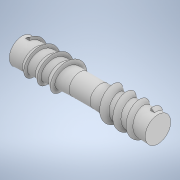
# Autodesk Inventor part: rolinho
Saved by Autodesk Inventor 2020 (Build 240168000, 168)
## iProperties
Created: 2021-06-17
Part Number: rolinho
Material: Generic
Document SubType Name: Modeling
Designer: Acer
Density: 1 g/cm^3
Appearance: Default
Author: Acer
Autodesk Inventor part; units mm, degrees
ref_plane "YZ Plane" through (0, 0, 0) normal (1, 0, 0) x (0, 1, 0)
ref_plane "XZ Plane" through (0, 0, 0) normal (0, 1, 0) x (-1, 0, 0)
ref_plane "XY Plane" through (0, 0, 0) normal (0, 0, 1) x (1, 0, 0)
sketch "Sketch1" plane through (0, 0, 0) normal (0, 0, 1) x (1, 0, 0)
  line L0 (0, 0) -> (36, 0)
  line L1 (36, 0) -> (36, 6.75)
  line L2 (36, 6.75) -> (0, 6.75)
  line L3 (0, 6.75) -> (0, 0)
  line L4 (5.5, 0) -> (5.5, 6.75)
  line L5 (0, 5.5) -> (5.5, 5.5)
  line L6 (5.5, 5.5) -> (36, 6.75)
  point P0 (0, 0)
  dimension "d0" = 36
  dimension "d1" = 6.75
  dimension "d2" = 0
  dimension "d3" = 6.75
  dimension "d19" = 5.5
  dimension "d20" = 5.5
  constraints: 14 end point, 4 point on line, 3 perpendicular, 2 parallel, 1 horizontal
  measures "d0" distance of L2.end L1.end
  measures "d1" distance of L1.end L0.end
  measures "d2" distance from line of L3 point (0, 0)
  measures "d3" distance from line of L2 point (0, 0)
  measures "d19" distance between parallel lines of L3 L4
  measures "d20" distance between parallel lines of L0 L5
revolve "Revolution1" add sketch "Sketch1" angle 360 about axis through (0, 0, 0) along (1, 0, 0) contours L3 L5 L4 L0 | L4 L6 L1 L0
sketch "Sketch2" plane through (0, 0, 0) normal (0, 0, 1) x (1, 0, 0)
  line L0 (36, -6.75) -> (36, 6.75) projected
  line L1 (0, -5.5) -> (0, 5.5)
  line L2 (36, -6.75) -> (36, 6.75) projected
  line L3 (36, 5) -> (31.9, 5)
  line L4 (31.9, 5) -> (31.9, 5.5)
  line L5 (31.9, 5.5) -> (36, 5.5)
  line L6 (36, 5.5) -> (36, 5)
  line L7 (31.8118, 5) -> (32.3232, 7.9)
  line L8 (31.9, 5.5) -> (33.5309, 5.5) construction
  line L9 (32.3232, 7.9) -> (36, 5.5)
  line L10 (31.9, 5) -> (31.8118, 5)
  line L11 (0, 0) -> (36, 0)
  line L12 (5.5, 5.5) -> (36, 6.75) projected
  line L13 (0, 5.5) -> (5.5, 5.5) projected
  line L14 (0, -5.5) -> (0, 5.5) projected
  dimension "d6" = 5
  dimension "d7" = 0.5
  dimension "d8" = 4.1
  dimension "d9" = 80
  dimension "d10" = 2.4
  constraints: 20 end point, 3 horizontal, 2 parallel, 2 point on line, 1 midpoint, 1 perpendicular
  measures "d6" distance from line of L11.start L3
  measures "d7" distance between parallel lines of L3 L5
  measures "d8" distance between parallel lines of L0 L4
  measures "d9" angle of L8 L7
  measures "d10" distance from line of L5 L7.end
coil "Coil1" sketch "Sketch2" operation add axis through (0, 0, 0) along (-1, 0, 0) pitch 7 turns 3.5 hand right contours L3 L4 L5 L0 | L5 L7 L12 L9 | L10 L7 L4 | L12 L7 L9
mirror "Mirror1" about plane through (0, 5.5, 0) normal (-1, 0, 0) of "Revolution1", "Coil1"
body "Solid1"
